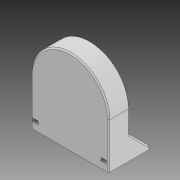
# Autodesk Inventor part: J1_idlebracket
Saved by Autodesk Inventor 2020 (Build 240168000, 168)
## iProperties
Created: 2021-03-20
Part Number: J1_idlebracket
Material: Generic
Document SubType Name: Modeling
Designer: DDeGo
Density: 1 g/cm^3
Appearance: Default
Author: DDeGo
Autodesk Inventor part; units mm, degrees
ref_plane "YZ Plane" through (0, 0, 0) normal (1, 0, 0) x (0, 1, 0)
ref_plane "XZ Plane" through (0, 0, 0) normal (0, 1, 0) x (-1, 0, 0)
sketch "Sketch1" plane through (0, 0, 0) normal (0, 0, 1) x (1, 0, 0)
  circle A0 centre (0, 0) radius 47.525
  arc A1 (60, 0) -> (-60, 0) centre (0, 0) ccw
  line L0 (-60, 0) -> (-60, -70)
  line L1 (-60, -70) -> (60, -70)
  line L2 (60, -70) -> (60, 0)
  dimension "d0" = 95.05
  dimension "d2" = 70
  dimension "d43" = 60
  constraints: 6 end point, 2 centre point, 2 coincident, 2 point on circle, 2 tangent, 2 vertical, 1 perpendicular
  measures "d0" diameter of A0
  measures "d2" distance from line of L1 point (0, 0)
  measures "d43" radius of A1
extrude "Extrusion1" add sketch "Sketch1" along normal blind 32.5
sketch "Sketch2" plane through (0, 0, 0) normal (0, 0, -1) x (-1, 0, 0)
  circle A0 centre (0, 0) radius 47.525 projected
  circle A1 centre (0, 0) radius 45.525
  dimension "d5" = 2
  constraints: 1 centre point, 1 coincident
  measures "d5" radial gap between concentric circles of A0 A1
extrude "Extrusion2" add sketch "Sketch2" against normal blind 1
sketch "Sketch3" plane through (0, 0, 32.5) normal (0, 0, 1) x (1, 0, 0)
  arc A0 (60, 0) -> (-60, 0) centre (0, 0) ccw construction
  line L0 (0, 0) -> (0, 55) construction
  circle A1 centre (0, 55) radius 2.6
  circle A2 centre (-52.3081, 16.9959) radius 2.6
  circle A3 centre (-32.3282, -44.4959) radius 2.6
  circle A4 centre (32.3282, -44.4959) radius 2.6
  circle A5 centre (52.3081, 16.9959) radius 2.6
  dimension "d8" = 5.2
  dimension "d9" = 55
  dimension "d12" = 360
  constraints: 5 centre point, 5 coincident, 2 end point, 1 vertical, 16 other
  measures "d8" diameter of A1
  measures "d9" distance of L0.start L0.end
extrude "Extrusion3" cut sketch "Sketch3" against normal through all
sketch "Sketch7" plane through (-60, -70, 0) normal (-1, 0, 0) x (0, 0, 1)
  line L0 (0, 0) -> (32.5, 0) projected
  line L1 (0, 0) -> (-30, 0)
  line L2 (-30, 0) -> (-30, 5)
  line L3 (0, 70) -> (0, 0) projected
  line L4 (-30, 5) -> (0, 35)
  line L5 (0, 0) -> (0, 35)
  dimension "d32" = 30
  dimension "d33" = 5
  dimension "d34" = 135
  constraints: 8 end point, 2 parallel, 1 horizontal, 1 midpoint
  measures "d32" distance of L0.start L1.end
  measures "d33" distance of L1.end L2.end
  measures "d34" angle of L2 L4
extrude "Extrusion7" add sketch "Sketch7" against normal blind 15
mirror "Mirror1" about plane through (0, 0, 0) normal (1, 0, 0) of "Extrusion7"
sketch "Sketch5" plane through (-60, -70, 0) normal (0, -1, 0) x (1, 0, 0)
  circle A0 centre (7.5, 25) radius 2.75
  circle A1 centre (112.5, 25) radius 2.75
  circle A2 centre (86.25, 7.5) radius 2.75
  circle A3 centre (33.75, 7.5) radius 2.75
  circle A4 centre (60, 25) radius 2.75
  line L0 (7.5, 25) -> (60, 25) construction
  line L1 (60, 25) -> (112.5, 25) construction
  line L2 (86.25, 7.5) -> (33.75, 7.5) construction
  line L3 (60, 25) -> (60, 7.5) construction
  line L4 (60, 7.5) -> (60, 0) construction
  line L5 (0, 0) -> (120, 0) construction
  line L6 (0, 32.5) -> (120, 32.5) construction
  line L7 (0, 0) -> (0, 32.5) construction
  line L8 (33.75, 25) -> (33.75, 7.5) construction
  line L9 (0, -30) -> (15, -30) construction
  line L10 (7.5, -30) -> (7.5, -20) construction
  line L11 (120, -30) -> (105, -30) construction
  line L12 (112.5, -30) -> (112.5, -20) construction
  line L13 (112.5, -20) -> (7.5, -20) construction
  circle A5 centre (7.5, -20) radius 2.75
  circle A6 centre (112.5, -20) radius 2.75
  line L14 (112.5, -20) -> (112.5, 25) construction
  line L15 (120, -30) -> (120, 32.5) projected
  dimension "d16" = 5.5
  dimension "d17" = 7.5
  dimension "d18" = 7.5
  dimension "d37" = 10
  dimension "d39" = 17.5
  dimension "d45" = 52.5
  dimension "d46" = 45
  dimension "d47" = 7.5
  constraints: 20 end point, 7 centre point, 6 equal radius, 6 vertical, 4 midpoint, 3 horizontal, 2 coincident, 1 collinear, 1 perpendicular
  measures "d16" diameter of A0
  measures "d17" distance between parallel lines of L5 L2
  measures "d18" distance between parallel lines of L6 L0
  measures "d37" distance of L10.start L10.end
  measures "d39" distance of L8.start L2.end
  measures "d45" distance of L0.end L1.end
  measures "d46" distance of L14.start L1.end
  measures "d47" distance between parallel lines of L15 L14
extrude "Extrusion4" cut sketch "Sketch5" against normal blind 18
ref_plane "Work Plane1" through (-60, -55, 0) normal (0, -1, 0) x (1, 0, 0)
sketch "Sketch6" plane through (-60, -55, 0) normal (0, -1, 0) x (1, 0, 0)
  circle A0 centre (112.5, 25) radius 2.75 projected
  circle A1 centre (60, 25) radius 2.75 projected
  circle A2 centre (33.75, 7.5) radius 2.75 projected
  line L0 (112.5, 29.7343) -> (116.6, 27.3671) construction
  line L1 (116.6, 27.3671) -> (116.6, 22.6329)
  line L2 (116.6, 22.6329) -> (112.5, 20.2657)
  line L3 (112.5, 20.2657) -> (108.4, 22.6329)
  line L4 (108.4, 22.6329) -> (108.4, 27.3671)
  line L5 (108.4, 27.3671) -> (112.5, 29.7343) construction
  line L6 (60, 29.7343) -> (64.1, 27.3671)
  line L7 (64.1, 27.3671) -> (64.1, 22.6329)
  line L8 (64.1, 22.6329) -> (60, 20.2657)
  line L9 (60, 20.2657) -> (55.9, 22.6329)
  line L10 (55.9, 22.6329) -> (55.9, 27.3671)
  line L11 (55.9, 27.3671) -> (60, 29.7343)
  circle A3 centre (33.75, 7.5) radius 2.75 projected
  line L12 (33.75, 2.7657) -> (29.65, 5.1329) construction
  line L13 (29.65, 5.1329) -> (29.65, 9.8671)
  line L14 (29.65, 9.8671) -> (33.75, 12.2343)
  line L15 (33.75, 12.2343) -> (37.85, 9.8671)
  line L16 (37.85, 9.8671) -> (37.85, 5.1329)
  line L17 (37.85, 5.1329) -> (33.75, 2.7657) construction
  circle A4 centre (86.25, 7.5) radius 2.75 projected
  line L18 (86.25, 2.7657) -> (82.15, 5.1329) construction
  line L19 (82.15, 5.1329) -> (82.15, 9.8671)
  line L20 (82.15, 9.8671) -> (86.25, 12.2343)
  line L21 (86.25, 12.2343) -> (90.35, 9.8671)
  line L22 (90.35, 9.8671) -> (90.35, 5.1329)
  line L23 (90.35, 5.1329) -> (86.25, 2.7657) construction
  circle A5 centre (7.5, 25) radius 2.75 projected
  line L24 (7.5, 20.2657) -> (3.4, 22.6329)
  line L25 (3.4, 22.6329) -> (3.4, 27.3671)
  line L26 (3.4, 27.3671) -> (7.5, 29.7343) construction
  line L27 (7.5, 29.7343) -> (11.6, 27.3671) construction
  line L28 (11.6, 27.3671) -> (11.6, 22.6329)
  line L29 (11.6, 22.6329) -> (7.5, 20.2657)
  line L30 (116.6, 27.3671) -> (116.6, 35.5137)
  line L31 (116.6, 35.5137) -> (108.4, 35.5137)
  line L32 (108.4, 35.5137) -> (108.4, 27.3671)
  line L33 (90.35, 5.1329) -> (90.35, -3.3085)
  line L34 (90.35, -3.3085) -> (82.15, -3.3085)
  line L35 (82.15, -3.3085) -> (82.15, 5.1329)
  line L36 (37.85, 5.1329) -> (37.85, -3.965)
  line L37 (37.85, -3.965) -> (29.65, -3.965)
  line L38 (29.65, -3.965) -> (29.65, 5.1329)
  line L39 (12.475, 1) -> (107.525, 1) projected
  line L40 (11.6, 27.3671) -> (11.6, 33.5607)
  line L41 (11.6, 33.5607) -> (3.4, 33.5607)
  line L42 (3.4, 33.5607) -> (3.4, 27.3671)
  circle A6 centre (112.5, -20) radius 2.75 projected
  circle A7 centre (112.5, -20) radius 2.75 projected
  circle A8 centre (7.5, -20) radius 2.75 projected
  line L43 (112.5, -24.7343) -> (108.4, -22.3671)
  line L44 (108.4, -22.3671) -> (108.4, -17.6329)
  line L45 (108.4, -17.6329) -> (112.5, -15.2657)
  line L46 (112.5, -15.2657) -> (116.6, -17.6329)
  line L47 (116.6, -17.6329) -> (116.6, -22.3671)
  line L48 (116.6, -22.3671) -> (112.5, -24.7343)
  line L49 (7.5, -24.7343) -> (3.4, -22.3671)
  line L50 (3.4, -22.3671) -> (3.4, -17.6329)
  line L51 (3.4, -17.6329) -> (7.5, -15.2657)
  line L52 (7.5, -15.2657) -> (11.6, -17.6329)
  line L53 (11.6, -17.6329) -> (11.6, -22.3671)
  line L54 (11.6, -22.3671) -> (7.5, -24.7343)
  point P0 (60, 0)
  point P1 (60, 25)
  point P2 (33.75, 7.5)
  point P3 (7.5, 25)
  point P4 (37.85, 1)
  point P5 (29.65, 1)
  point P6 (90.35, 1)
  point P7 (82.15, 1)
  point P8 (7.5, -20)
  dimension "d23" = 8.2
  constraints: 108 end point, 11 vertical, 7 coincident, 6 equal length, 5 perpendicular, 3 collinear, 91 other
  measures "d23" distance between parallel lines of L4 L1
extrude "Extrusion5" cut sketch "Sketch6" along normal blind 4.5 contours A1 | L1 L2 L3 L4 L32 L31 L30 | L6 L7 L8 L9 L10 L11 | L35 L19 L20 L21 L22 L33 L39 | L39 L33 L34 L35 | L13 L14 L15 L16 L36 L39 L38 | L39 L36 L37 L38 | L24 L25 L42 L41 L40 L28 L29 | L43 L44 L45 L46 L47 L48 | L49 L50 L51 L52 L53 L54
extrude "Extrusion6" cut sketch "Sketch6" against normal blind 20.75 contours A1 | L6 L7 L8 L9 L10 L11 | L43 L44 L45 L46 L47 L48 | L49 L50 L51 L52 L53 L54
fillet "Fillet1" radius 2 1 edges at (-47.525, 0, 32.5)
chamfer "Chamfer1" distance 2 angle 45 10 edges at (0, 60, 32.5) (-60, -35, 32.5) (60, -35, 32.5) (0, 60, 0) (-60, -17.5, 0) (60, -17.5, 0) (-60, -50, -15) (-45, -50, -15) (45, -50, -15) (60, -50, -15)
fillet "Fillet2" radius 5 4 edges at (-45, -53.9142, 0) (45, -53.9142, 0) (52.5, -35, 0) (-52.5, -35, 0)
chamfer "Chamfer2" distance 2 angle 45 1 edges at (-47.525, 0, 1)
sketch "Sketch9" plane through (0, 0, 32.5) normal (0, 0, 1) x (1, 0, 0)
  circle A0 centre (0, 0) radius 47.525 projected
  circle A1 centre (0, 0) radius 47.525 projected
extrude "Extrusion8" cut sketch "Sketch9" against normal through all
sketch "Sketch10" plane through (0, 0, 32.5) normal (0, 0, 1) x (1, 0, 0)
  circle A0 centre (-32.3282, -44.4959) radius 2.6 projected
  circle A1 centre (-52.3081, 16.9959) radius 2.6 projected
  circle A2 centre (0, 55) radius 2.6 projected
  circle A3 centre (52.3081, 16.9959) radius 2.6 projected
  circle A4 centre (32.3282, -44.4959) radius 2.6 projected
  point P0 (0, 0)
extrude "Extrusion9" add sketch "Sketch10" against normal up to surface (32.5 mm away)
sketch "Sketch11" plane through (0, 0, 32.5) normal (0, 0, 1) x (1, 0, 0)
  circle A0 centre (0, 0) radius 49.525 projected
extrude "Extrusion10" add sketch "Sketch11" against normal blind 3
equation "\"d17\" = d47"
equation "\"d18\" = d47"
body "Solid1"
